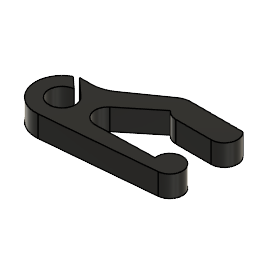
baghookthing (Autodesk Fusion 360 design; units mm, degrees)
Autodesk Fusion 360 part; units mm, degrees
note: some values were not read from the file. Set by a fixed rule: which sketch regions a step uses.
sketch "Sketch1" plane through (0, 0, 0) normal (0, 0, 1) x (1, 0, 0)
  arc A0 (0.5431, -5.9754) -> (-6, -0.0009) centre (0, 0) ccw
  line L0 (-57.082, 11.9268) -> (-52.7612, 7.9603)
  line L1 (-54.7452, 12.4965) -> (-48.0478, 6.3484)
  arc A1 (-52.7612, 7.9603) -> (-48.0478, 6.3484) centre (-52.2429, 1.7784) ccw
  line L2 (-51.1115, -10.6703) -> (0.5431, -5.9754)
  arc A2 (-58.0724, 12.8359) -> (-51.1115, -10.6703) centre (-52.2429, 1.7784) ccw
  line L3 (-54.7452, 12.4965) -> (-56.1222, 13.7606)
  line L4 (-52.7612, 7.9603) -> (-58.0724, 12.8359)
  line L5 (-33.1127, -1.7115) -> (-5.9176, -0.9908)
  arc A3 (-37.0573, 8.9414) -> (-33.1127, -1.7115) centre (-33.2717, 4.2864) ccw
  arc A4 (0.5431, -5.9754) -> (-5.9176, -0.9908) centre (0, 0) ccw
  line L6 (-37.0573, 8.9414) -> (-21.3737, 21.6961)
  line L7 (0, 0) -> (-3.6487, 4.7631)
  arc A5 (-57.5185, 13.1106) -> (-51.1115, -10.6703) centre (-52.2429, 1.7784) ccw
  line L8 (-26.4923, 27.5542) -> (-41.8134, 16.7543)
  line L9 (-50.8798, 13.8799) -> (-55.8659, 13.8799)
  line L10 (-56.1222, 13.7606) -> (-55.8659, 13.8799)
  arc A6 (-50.8798, 13.8799) -> (-41.8134, 16.7543) centre (-50.8798, 29.6161) ccw
  line L11 (-16.5939, 19.3899) -> (0, 19.3899)
  arc A7 (0, 19.3899) -> (4.2678, 30.1155) centre (0, 25.6018) ccw
  line L12 (-26.4923, 27.5542) -> (-25.0264, 28.5876)
  arc A8 (-21.3737, 21.6961) -> (-16.4556, 19.3899) centre (-16.5058, 25.6799) ccw
  arc A9 (-21.3737, 21.6961) -> (-16.4556, 19.3899) centre (-16.5248, 25.6395) ccw
  arc A10 (0, 19.3899) -> (4.2678, 30.1155) centre (0, 25.6018) ccw
  line L13 (-20.2069, 30.1155) -> (4.2678, 30.1155)
  arc A11 (-20.2069, 30.1155) -> (-25.0264, 28.5876) centre (-20.2069, 21.7505) ccw
  dimension "d6" = 12
  dimension "d8" = 12.5
  dimension "d10" = 2
  dimension "d13" = 25
  dimension "d15" = 12
  dimension "d20" = 8.365
  constraint coincident A0.centre A4.centre
  constraint parallel L0 L1
  constraint tangent L1 A1
  constraint tangent A2 L10
  constraint tangent L2 A2
  constraint tangent A0 L2
  constraint parallel L1 L3
  constraint parallel L0 L4
  constraint tangent L5 A3
  constraint concentric A0 A4
  constraint coincident A0.end A4
  constraint coincident A1.centre A2.centre
  constraint tangent A3 L6
  constraint coincident A0 L7.end
  constraint concentric A2 A5
  constraint coincident A5.start L10
  constraint horizontal L9
  constraint tangent L8 A6
  constraint tangent L9 A6
  constraint tangent L11 A7
  constraint concentric A7 A10
  constraint parallel L8 L12
  constraint coincident L11.start A9
  constraint coincident L11 A8.end
  constraint horizontal L13
  constraint tangent L13 A11
  constraint tangent L12 A11
  measures "d6" diameter of A0
  measures "d8" diameter of A9
  measures "d10" distance of L0 L1
  measures "d13" diameter of A2
  measures "d15" diameter of A3
  measures "d20" radius of A11
extrude "Extrude1" add sketch "Sketch1" along normal blind 10
extrude "Extrude2" add sketch "Sketch1" along normal up to surface (10 mm away)
